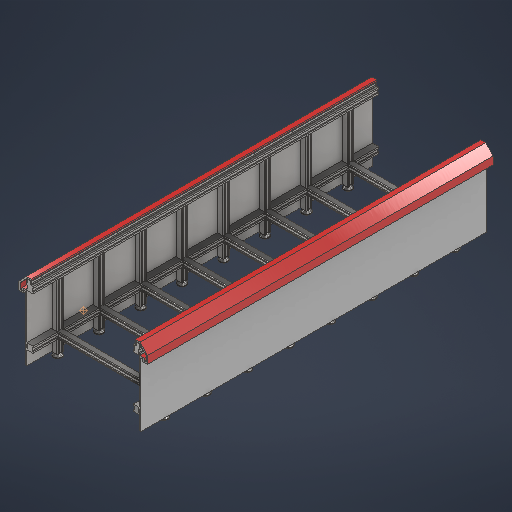
# Autodesk Inventor part: CONVEYOR STRUCTURE-03
Saved by Autodesk Inventor 2025 (Build 290162000, 162)
## iProperties
Created: 2024-05-06
Part Number: CONVEYOR STRUCTURE-03
Material: Generic
Document SubType Name: Modeling
Designer: zulet
Density: 1 g/cm^3
Appearance: Steel - Polished
conveyorWidth: 1500,000 mm
conveyorLength: 5000,000 mm
rollerSeparation: 110,000 mm
Author: zulet
Autodesk Inventor part; units mm, degrees
ref_plane "XZ Plane" through (0, 0, 0) normal (0, 1, 0) x (-1, 0, 0)
ref_plane "XY Plane" through (0, 0, 0) normal (0, 0, 1) x (1, 0, 0)
ref_plane "Work Plane1" through (770, 0, 0) normal (1, 0, 0) x (0, 1, 0)
sketch "Sketch1" plane through (770, 0, 0) normal (1, 0, 0) x (0, 1, 0)
  line L0 (0, 0) -> (-55, 0)
  line L1 (-55, 0) -> (-55, -5000)
  line L2 (-55, -5000) -> (0, -5000)
  line L3 (0, -5000) -> (0, 0)
  line L4 (-55, 0) -> (-145, 0)
  line L5 (-145, 0) -> (-145, -5000)
  line L6 (-145, -5000) -> (-55, -5000)
  line L7 (-55, -5000) -> (-55, 0)
  line L8 (-145, -355) -> (-1090, -355)
  line L9 (-1090, -355) -> (-1090, -445)
  line L10 (-1090, -445) -> (-145, -445)
  line L11 (-145, -445) -> (-145, -355)
  line L12 (-890, 0) -> (-800, 0)
  line L13 (-800, 0) -> (-800, -5000)
  line L14 (-800, -5000) -> (-890, -5000)
  line L15 (-890, -5000) -> (-890, 0)
  circle A0 centre (-20, -55) radius 7.5 construction
  line L16 (-5, -5) -> (-50, -5)
  line L17 (-50, -5) -> (-50, -4995)
  line L18 (-50, -4995) -> (-5, -4995)
  line L19 (-5, -4995) -> (-5, -5)
  line L20 (-1090, -400) -> (-145, -400) construction
  line L21 (-145, -955) -> (-1090, -955)
  line L22 (-1090, -1045) -> (-145, -1045)
  line L23 (-1090, -1000) -> (-145, -1000) construction
  line L24 (-1090, -955) -> (-1090, -1045)
  line L25 (-145, -1045) -> (-145, -955)
  line L26 (-145, -1555) -> (-1090, -1555)
  line L27 (-1090, -1645) -> (-145, -1645)
  line L28 (-1090, -1600) -> (-145, -1600) construction
  line L29 (-1090, -1555) -> (-1090, -1645)
  line L30 (-145, -1645) -> (-145, -1555)
  line L31 (-145, -2155) -> (-1090, -2155)
  line L32 (-1090, -2245) -> (-145, -2245)
  line L33 (-1090, -2200) -> (-145, -2200) construction
  line L34 (-1090, -2155) -> (-1090, -2245)
  line L35 (-145, -2245) -> (-145, -2155)
  line L36 (-145, -2755) -> (-1090, -2755)
  line L37 (-1090, -2845) -> (-145, -2845)
  line L38 (-1090, -2800) -> (-145, -2800) construction
  line L39 (-1090, -2755) -> (-1090, -2845)
  line L40 (-145, -2845) -> (-145, -2755)
  line L41 (-145, -3355) -> (-1090, -3355)
  line L42 (-1090, -3445) -> (-145, -3445)
  line L43 (-1090, -3400) -> (-145, -3400) construction
  line L44 (-1090, -3355) -> (-1090, -3445)
  line L45 (-145, -3445) -> (-145, -3355)
  line L46 (-145, -3955) -> (-1090, -3955)
  line L47 (-1090, -4045) -> (-145, -4045)
  line L48 (-1090, -4000) -> (-145, -4000) construction
  line L49 (-1090, -3955) -> (-1090, -4045)
  line L50 (-145, -4045) -> (-145, -3955)
  line L51 (-145, -4555) -> (-1090, -4555)
  line L52 (-1090, -4645) -> (-145, -4645)
  line L53 (-1090, -4600) -> (-145, -4600) construction
  line L54 (-1090, -4555) -> (-1090, -4645)
  line L55 (-145, -4645) -> (-145, -4555)
  point P0 (-800, -445)
  point P1 (-145, -445)
  point P2 (-145, -955)
  point P3 (-800, -955)
  point P4 (-800, -1045)
  point P5 (-145, -1045)
  point P6 (-145, -1555)
  point P7 (-800, -1555)
  point P8 (-800, -1645)
  point P9 (-145, -1645)
  point P10 (-145, -2155)
  point P11 (-800, -2155)
  point P12 (-800, -2245)
  point P13 (-145, -2245)
  point P14 (-145, -2755)
  point P15 (-800, -2755)
  point P16 (-800, -355)
  point P17 (-890, -355)
  point P18 (-890, -445)
  point P19 (-890, -955)
  point P20 (-890, -1045)
  point P21 (-890, -1555)
  point P22 (-890, -1645)
  point P23 (-890, -2155)
  point P24 (-890, -2245)
  point P25 (-890, -2755)
  point P26 (-890, -2845)
  point P27 (-800, -2845)
  point P28 (-145, -2845)
  point P29 (-55, -5000)
  point P30 (-20, -165)
  point P31 (-20, -275)
  point P32 (-20, -385)
  point P33 (-20, -495)
  point P34 (-20, -605)
  point P35 (-20, -715)
  point P36 (-20, -825)
  point P37 (-20, -935)
  point P38 (-20, -1045)
  point P39 (-20, -1155)
  point P40 (-20, -1265)
  point P41 (-20, -1375)
  point P42 (-20, -1485)
  point P43 (-20, -1595)
  point P44 (-20, -1705)
  point P45 (-20, -1815)
  point P46 (-20, -1925)
  point P47 (-20, -2035)
  point P48 (-20, -2145)
  point P49 (-20, -2255)
  point P50 (-20, -2365)
  point P51 (-20, -2475)
  point P52 (-20, -2585)
  point P53 (-20, -2695)
  point P54 (-20, -2805)
  point P55 (-20, -2915)
  point P56 (-20, -3025)
  point P57 (-20, -3135)
  point P58 (-20, -3245)
  point P59 (-20, -3355)
  point P60 (-20, -3465)
  point P61 (-20, -3575)
  point P62 (-20, -3685)
  point P63 (-20, -3795)
  point P64 (-20, -3905)
  point P65 (-20, -4015)
  point P66 (-20, -4125)
  point P67 (-20, -4235)
  point P68 (-20, -4345)
  point P69 (-20, -4455)
  point P70 (-20, -4565)
  point P71 (-20, -4675)
  point P72 (-20, -4785)
  point P73 (-20, -4895)
  dimension "d1" = 15
  dimension "d2" = 55
  dimension "d3" = 5000
  dimension "d11" = 20
  dimension "d12" = 55
  dimension "d13" = 5
  dimension "d14" = 1090
  dimension "d15" = 90
  dimension "d16" = 90
  dimension "d17" = 90
  dimension "d18" = 200
  dimension "d21" = 600
  dimension "d84" = 400
  dimension "d104" = 110
  constraints: 112 end point, 10 parallel, 5 perpendicular, 4 horizontal, 3 collinear, 2 midpoint, 2 vertical, 1 centre point, 1 coincident, 1 point on line, 124 other
  measures "d1" diameter of A0
  measures "d2" distance from line of L0 A0.centre
  measures "d3" distance of L2.end L0.start
  measures "d11" distance from line of L3 A0.centre
  measures "d12" distance of L0.start L0.end
  measures "d13" distance between parallel lines of L3 L19
  measures "d14" distance between parallel lines of L9 L3
  measures "d15" distance of L0.end L4.end
  measures "d16" distance of L8.end L9.end
  measures "d17" distance of L12.start L12.end
  measures "d18" distance between parallel lines of L15 L9
  measures "d21" distance of L8.start L21.start
  measures "d84" distance between parallel lines of L4 L20
  measures "d104" distance of point (-20, -55) point (-20, -165)
extrude "Extrusion1" add sketch "Sketch1" along normal mid plane 90 contours L1 L6 L5 L4 | L13 L10 L15 L8 | L8 L15 L12 L13 | L52 L15 L51 L13 | L13 L14 L15 L52 | L13 L21 L15 L10 | L51 L15 L47 L13 | L13 L22 L15 L21 | L47 L15 L46 L13 | L13 L26 L15 L22 | L46 L15 L42 L13 | L13 L27 L15 L26 | L42 L15 L41 L13 | L13 L31 L15 L27 | L41 L15 L37 L13 | L13 L32 L15 L31 | L37 L15 L36 L13 | L13 L36 L15 L32
extrude "Extrusion2" add sketch "Sketch1" along normal blind 45 and the other way blind 18 contours L3 L2 L1 L0
extrude "Extrusion3" add sketch "Sketch1" along normal blind 35 contours L19 L18 L17 L16
sketch "Sketch2" plane through (725, 0, 0) normal (-1, 0, 0) x (0, 0, 1)
  line L0 (-5000, -55) -> (-5000, -145) projected
  line L1 (0, -145) -> (0, -55) projected
  line L2 (0, -890) -> (0, -800) projected
  line L3 (-5000, -800) -> (-5000, -890) projected
  line L4 (-5000, -77.5) -> (0, -77.5)
  line L5 (0, -77.5) -> (0, -122.5)
  line L6 (0, -122.5) -> (-5000, -122.5)
  line L7 (-5000, -122.5) -> (-5000, -77.5)
  line L8 (-5000, -822.5) -> (0, -822.5)
  line L9 (0, -822.5) -> (0, -867.5)
  line L10 (0, -867.5) -> (-5000, -867.5)
  line L11 (-5000, -867.5) -> (-5000, -822.5)
  line L12 (0, -800) -> (-5000, -800) projected
  line L13 (-5000, -890) -> (0, -890) projected
  point P0 (0, 0)
  point P1 (-275, -800)
  point P2 (-275, -890)
  point P3 (0, -822.5)
  point P4 (0, -77.5)
  dimension "d36" = 45
  dimension "d37" = 22.5
  dimension "d38" = 22.5
  dimension "d39" = 45
  dimension "d40" = 22.5
  dimension "d41" = 22.5
  constraints: 16 end point, 4 parallel, 4 point on line, 2 horizontal, 2 perpendicular
  measures "d36" distance between parallel lines of L4 L6
  measures "d37" distance from line of L1.end L4
  measures "d38" distance from line of L6 L1.start
  measures "d39" distance between parallel lines of L10 L8
  measures "d40" distance between parallel lines of L12 L8
  measures "d41" distance between parallel lines of L13 L10
extrude "Extrusion4" cut sketch "Sketch2" against normal blind 15 contours L4 L1 L6 L0 | L10 L3 L8 L2
mirror "Mirror1" about plane through (770, 0, 0) normal (1, 0, 0) of "Extrusion4"
extrude "Extrusion10" add sketch "Sketch1" along normal mid plane 90 contours L5 L10 L13 L8 | L15 L10 L9 L8
sketch "Sketch3" plane through (725, 0, 0) normal (-1, 0, 0) x (0, 0, 1)
  line L0 (-445, -800) -> (-445, -145) construction
  line L1 (-445, -145) -> (-355, -145) construction
  line L2 (-445, -800) -> (-355, -800) construction
  line L3 (0, -890) -> (-5000, -890) construction
  line L4 (-445, -890) -> (-355, -890) construction
  line L5 (-422.5, -145) -> (-377.5, -145)
  line L6 (-377.5, -145) -> (-377.5, -800)
  line L7 (-377.5, -800) -> (-422.5, -800)
  line L8 (-422.5, -800) -> (-422.5, -145)
  line L9 (-369.5668, -1090) -> (-291.7701, -1090)
  line L10 (-422.5, -890) -> (-377.5, -890)
  line L11 (-377.5, -890) -> (-377.5, -1090)
  line L12 (-377.5, -1090) -> (-422.5, -1090)
  line L13 (-422.5, -1090) -> (-422.5, -890)
  line L14 (-355, -800) -> (-355, -145) construction
  line L15 (-445, -145) -> (-445, -800) projected
  line L16 (-355, -800) -> (-355, -145) projected
  line L17 (-445, -1090) -> (-355, -1090) projected
  point P0 (0, 0)
  point P1 (-342.5, -1090)
  dimension "d44" = 45
  dimension "d45" = 22.5
  dimension "d46" = 22.5
  constraints: 28 end point, 6 point on line, 4 collinear, 4 parallel, 3 horizontal, 2 perpendicular
  measures "d44" distance between parallel lines of L8 L6
  measures "d45" distance between parallel lines of L14 L6
  measures "d46" distance between parallel lines of L0 L8
extrude "Extrusion5" cut sketch "Sketch3" against normal blind 15
fillet "Fillet1" radius 10 4 edges at (725, -472.5, -355) (725, -472.5, -445) (725, -990, -445) (725, -990, -355)
mirror "Mirror2" about plane through (770, 0, 0) normal (1, 0, 0) of "Extrusion5", "Fillet1"
sketch "Sketch5" plane through (770, 0, 0) normal (1, 0, 0) x (0, 1, 0)
  line L0 (-1090, -377.5) -> (-1090, -422.5)
  line L1 (-1090, -400) -> (-1140, -400)
  line L2 (-1140, -400) -> (-1140, -460)
  line L3 (-1140, -460) -> (-1130, -460)
  line L4 (-1130, -460) -> (-1090, -422.5)
  line L5 (-1090, -377.5) -> (-1090, -422.5) projected
  point P0 (0, 0)
  dimension "d56" = 50
  dimension "d57" = 60
  dimension "d58" = 10
  constraints: 10 end point, 2 horizontal, 1 midpoint, 1 vertical
  measures "d56" distance of L1.start L1.end
  measures "d57" distance of L1.end L2.end
  measures "d58" distance of L2.end L3.end
revolve "Revolution1" add sketch "Sketch5" angle 360 about axis through (770, -1090, -400) along (0, -1, 0)
sketch "Sketch6" plane through (725, 0, 0) normal (-1, 0, 0) x (0, 0, 1)
  line L0 (-445, -145) -> (-445, -800)
  line L1 (-355, -1090) -> (-355, -890)
  line L2 (-435, -800) -> (-365, -800)
  line L3 (-355, -810) -> (-355, -880)
  line L4 (-365, -890) -> (-435, -890)
  line L5 (-445, -880) -> (-445, -810)
  line L6 (0, -822.5) -> (-5000, -822.5) construction
  line L7 (0, -867.5) -> (-5000, -867.5) construction
  line L8 (-445, -822.5) -> (-430, -822.5)
  line L9 (-430, -822.5) -> (-430, -867.5)
  line L10 (-430, -867.5) -> (-445, -867.5)
  line L11 (-445, -867.5) -> (-445, -822.5)
  line L12 (-355, -822.5) -> (-370, -822.5)
  line L13 (-370, -822.5) -> (-370, -867.5)
  line L14 (-370, -867.5) -> (-355, -867.5)
  line L15 (-355, -867.5) -> (-355, -822.5)
  arc A0 (-435, -800) -> (-445, -810) centre (-435, -810) ccw
  arc A1 (-355, -810) -> (-365, -800) centre (-365, -810) ccw
  arc A2 (-365, -890) -> (-355, -880) centre (-365, -880) ccw
  arc A3 (-445, -880) -> (-435, -890) centre (-435, -880) ccw
  line L16 (-445, -145) -> (-445, -800) projected
  line L17 (-355, -1090) -> (-355, -890) projected
  point P0 (0, 0)
  dimension "d60" = 15
  dimension "d61" = 15
  dimension "d62" = 10
  constraints: 28 end point, 10 point on line, 8 point on circle, 8 tangent, 6 parallel, 4 centre point, 3 equal radius, 3 horizontal, 3 perpendicular
  measures "d60" distance between parallel lines of L5 L9
  measures "d61" distance between parallel lines of L13 L3
  measures "d62" radius of A0
extrude "Extrusion7" add sketch "Sketch6" along normal up to surface (725 mm away) contours L2 A1 L3 L12 L13 L14 A2 L4 A3 L5 L10 L9 L8 A0
pattern_linear "Rectangular Pattern2" count 8 spacing 600 along (0, 0, -1) of "Extrusion10", "Extrusion5", "Fillet1", "Mirror2", "Revolution1", "Extrusion7"
sketch "Sketch7" plane through (815, 0, 0) normal (1, 0, 0) x (0, 0, -1)
  line L0 (0, -122.5) -> (0, -145) projected
  line L1 (0, -145) -> (5000, -145)
  line L2 (5000, -145) -> (5000, -1090)
  line L3 (5000, -1090) -> (0, -1090)
  line L4 (0, -1090) -> (0, -145)
  point P0 (0, 0)
  dimension "d68" = 5000
  dimension "d87" = 945
  constraints: 8 end point, 2 parallel, 1 horizontal, 1 perpendicular
  measures "d68" distance of L2.end L3.end
  measures "d87" distance of L3.end L0.end
extrude "Extrusion8" add sketch "Sketch7" along normal blind 20
sketch "Sketch8" plane through (740, -867.5, 0) normal (0, 0, 1) x (1, 0, 0)
  line L0 (95, 722.5) -> (95, -222.5) projected
  line L1 (95, 722.5) -> (145, 722.5)
  line L2 (145, 722.5) -> (145, 687.5)
  line L3 (145, 687.5) -> (170, 687.5)
  line L4 (170, 687.5) -> (170, 769.6752)
  line L5 (170, 769.6752) -> (75, 872.5)
  line L6 (75, 872.5) -> (12, 872.5)
  line L7 (12, 872.5) -> (12, 892.5)
  line L8 (12, 892.5) -> (83.7513, 892.5)
  line L9 (83.7513, 892.5) -> (190, 777.5)
  line L10 (190, 777.5) -> (190, 667.5)
  line L11 (190, 667.5) -> (125, 667.5)
  line L12 (125, 667.5) -> (125, 702.5)
  line L13 (125, 702.5) -> (95, 702.5)
  line L14 (12, 867.5) -> (75, 867.5) construction
  line L15 (12, 867.5) -> (12, 872.5) construction
  line L16 (75, 790) -> (75, 867.5) construction
  line L17 (75, 867.5) -> (75, 872.5) construction
  point P0 (-740, 867.5)
  point P1 (157.5, 687.5)
  dimension "d71" = 20
  dimension "d72" = 20
  dimension "d73" = 20
  dimension "d74" = 20
  dimension "d75" = 20
  dimension "d76" = 20
  dimension "d77" = 50
  dimension "d78" = 65
  dimension "d79" = 15
  dimension "d80" = 5
  dimension "d81" = 110
  constraints: 30 end point, 8 perpendicular, 3 parallel, 2 vertical, 1 horizontal, 1 midpoint, 1 point on line
  measures "d71" distance between parallel lines of L13 L1
  measures "d72" distance between parallel lines of L2 L12
  measures "d73" distance between parallel lines of L11 L3
  measures "d74" distance between parallel lines of L10 L4
  measures "d75" distance between parallel lines of L9 L5
  measures "d76" distance between parallel lines of L8 L6
  measures "d77" distance between parallel lines of L0 L2
  measures "d78" distance of L10.end L11.end
  measures "d79" distance from line of point (157.5, 687.5) L13
  measures "d80" distance of L14.start L6.end
  measures "d81" distance from line of L11 L9.end
extrude "Extrusion9" add sketch "Sketch8" against normal blind 5000
hole "Hole1" at (770, -20, -55) direction (1, 0, 0) diameter 15 depth 10
pattern_sketch "Sketch Driven Pattern1" of "Hole1" from (770, -20, -55) copies at (770, -20, -165) at (770, -20, -275) at (770, -20, -385) at (770, -20, -495) at (770, -20, -605) at (770, -20, -715) at (770, -20, -825) at (770, -20, -935) at (770, -20, -1045) at (770, -20, -1155) at (770, -20, -1265) at (770, -20, -1375) at (770, -20, -1485) at (770, -20, -1595) at (770, -20, -1705) at (770, -20, -1815) at (770, -20, -1925) at (770, -20, -2035) at (770, -20, -2145) at (770, -20, -2255) at (770, -20, -2365) at (770, -20, -2475) at (770, -20, -2585) at (770, -20, -2695) at (770, -20, -2805) at (770, -20, -2915) at (770, -20, -3025) at (770, -20, -3135) at (770, -20, -3245) at (770, -20, -3355) at (770, -20, -3465) at (770, -20, -3575) at (770, -20, -3685) at (770, -20, -3795) at (770, -20, -3905) at (770, -20, -4015) at (770, -20, -4125) at (770, -20, -4235) at (770, -20, -4345) at (770, -20, -4455) at (770, -20, -4565) at (770, -20, -4675) at (770, -20, -4785) at (770, -20, -4895)
mirror "Mirror4" about plane through (0, 0, 0) normal (1, 0, 0) of "Extrusion1", "Extrusion2", "Extrusion3", "Extrusion4", "Mirror1", "Extrusion10", "Extrusion5", "Fillet1", "Mirror2", "Revolution1", "Extrusion7", "Rectangular Pattern2", "Extrusion8", "Extrusion9", "Hole1", "Sketch Driven Pattern1"
sketch "Sketch11" plane through (752, 0, 0) normal (0, 0, 1) x (1, 0, 0)
  line L0 (0, -55) -> (0, 0) projected
  line L1 (0, 0) -> (-2, 0)
  line L2 (-2, 0) -> (-2, -4)
  line L3 (-2, -4) -> (0, -4)
  line L4 (0, -4) -> (0, 0)
  point P0 (-752, 0)
  dimension "d110" = 2
  dimension "d111" = 4
  constraints: 8 end point, 2 parallel, 1 horizontal, 1 perpendicular
  measures "d110" distance of L3.end L2.end
  measures "d111" distance of L2.end L1.end
extrude "Extrusion11" add sketch "Sketch11" against normal up to surface (5 mm away)
equation "\"d2\" = 0.5 * rollerSeparation"
equation "\"d3\" = conveyorLength"
equation "\"d16\" = d15"
equation "\"d17\" = d15"
equation "\"d28\" = d15"
equation "\"d30\" = 0.5 * d15"
equation "\"d36\" = 0.5 * d15"
equation "\"d37\" = d38"
equation "\"d39\" = 0.5 * d15"
equation "\"d40\" = d41"
equation "\"d44\" = 0.5 * d15"
equation "\"d45\" = d46"
equation "\"d65\" = 0.0166667 * conveyorLength"
equation "\"d68\" = conveyorLength"
equation "\"d72\" = d71"
equation "\"d73\" = d71"
equation "\"d74\" = d71"
equation "\"d75\" = d71"
equation "\"d76\" = d71"
equation "\"d82\" = conveyorLength"
equation "\"conveyorWidth\" = 1500"
equation "\"rollerSeparation\" = 110"
equation "\"conveyorLength\" = 5000"
equation "\"d19\" = 0.0166667 * conveyorLength"
body "Solid1"
